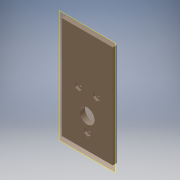
# Autodesk Inventor part: Motor cover lower
Saved by Autodesk Inventor 2019 (Build 230136000, 136)
## iProperties
Created: 2018-11-25
Part Number: Motor cover lower
Material: Generic
Document SubType Name: Modeling
Designer: Varga Daniel
Density: 1 g/cm^3
Appearance: Default
Author: Varga Daniel
Autodesk Inventor part; units mm, degrees
ref_plane "YZ Plane" through (0, 0, 0) normal (1, 0, 0) x (0, 1, 0)
ref_plane "XZ Plane" through (0, 0, 0) normal (0, 1, 0) x (-1, 0, 0)
ref_plane "Work Plane2" through (20, -5.2, 6) normal (0, 0, 1) x (1, 0, 0)
sketch "Sketch1" plane through (20, -5.2, 6) normal (0, 0, 1) x (1, 0, 0)
  line L0 (-33.75, 50) -> (16.25, 50)
  line L1 (16.25, 50) -> (16.25, -50)
  line L2 (16.25, -50) -> (-33.75, -50)
  line L3 (-33.75, -50) -> (-33.75, 50)
  line L4 (-33.75, 0) -> (16.25, 0) construction
  line L5 (-8.75, 50) -> (-8.75, -50) construction
  line L6 (-33.75, 0) -> (16.25, 0) construction
  circle A0 centre (-17.5, 0) radius 1.35
  circle A1 centre (0, 0) radius 1.35
  circle A2 centre (-8.75, -34.3) radius 1.35
  circle A3 centre (-8.75, -20.6) radius 7.25
  dimension "d0" = 50
  dimension "d1" = 100
  dimension "d15" = 2.7
  dimension "d16" = 2.7
  dimension "d17" = 2.7
  dimension "d18" = 14.5
  dimension "d19" = 17.5
  dimension "d20" = 20.6
  dimension "d21" = 34.3
  dimension "d22" = 15.7
  dimension "d23" = 16.25
  constraints: 14 end point, 6 midpoint, 4 centre point, 4 point on line, 2 parallel, 2 perpendicular, 1 horizontal
  measures "d0" distance between parallel lines of L3 L1
  measures "d1" distance between parallel lines of L2 L0
  measures "d15" diameter of A0
  measures "d16" diameter of A1
  measures "d17" diameter of A2
  measures "d18" diameter of A3
  measures "d19" distance of A1.centre A0.centre
  measures "d20" vertical distance of A3.centre A0.centre
  measures "d21" vertical distance of A2.centre A0.centre
  measures "d22" distance from line of A2.centre L2
  measures "d23" distance from line of A0.centre L3
extrude "Extrusion2" add sketch "Sketch1" against normal blind 4
sketch "Sketch2" plane through (20, -5.2, 6) normal (0, 0, 1) x (1, 0, 0)
  circle A0 centre (-8.75, -20.6) radius 7.25 construction
  circle A1 centre (-8.75, -34.3) radius 1.35 construction
  circle A2 centre (0, 0) radius 1.35 construction
  circle A3 centre (-17.5, 0) radius 1.35 construction
  line L0 (-33.75, 50) -> (16.25, 50) construction
  line L1 (-33.75, -50) -> (-33.75, 50) construction
  line L2 (16.25, -50) -> (-33.75, -50) construction
  line L3 (16.25, 50) -> (16.25, -50) construction
  line L4 (-14.4, -1.7898) -> (-17.5, -3.5796)
  line L5 (-17.5, -3.5796) -> (-20.6, -1.7898)
  line L6 (-20.6, -1.7898) -> (-20.6, 1.7898)
  line L7 (-20.6, 1.7898) -> (-17.5, 3.5796)
  line L8 (-17.5, 3.5796) -> (-14.4, 1.7898)
  line L9 (-14.4, 1.7898) -> (-14.4, -1.7898)
  line L10 (3.1, -1.7898) -> (0, -3.5796)
  line L11 (0, -3.5796) -> (-3.1, -1.7898)
  line L12 (-3.1, -1.7898) -> (-3.1, 1.7898)
  line L13 (-3.1, 1.7898) -> (0, 3.5796)
  line L14 (0, 3.5796) -> (3.1, 1.7898)
  line L15 (3.1, 1.7898) -> (3.1, -1.7898)
  line L16 (-5.65, -36.0898) -> (-8.75, -37.8796)
  line L17 (-8.75, -37.8796) -> (-11.85, -36.0898)
  line L18 (-11.85, -36.0898) -> (-11.85, -32.5102)
  line L19 (-11.85, -32.5102) -> (-8.75, -30.7204)
  line L20 (-8.75, -30.7204) -> (-5.65, -32.5102)
  line L21 (-5.65, -32.5102) -> (-5.65, -36.0898)
  line L22 (-33.75, -50) -> (-33.75, 50) projected
  point P0 (-20, 5.2)
  dimension "d26" = 6.2
  dimension "d27" = 6.2
  dimension "d28" = 6.2
  constraints: 36 end point, 3 coincident, 3 parallel, 39 other
  measures "d26" distance between parallel lines of L9 L6
  measures "d27" distance between parallel lines of L15 L12
  measures "d28" distance between parallel lines of L18 L21
extrude "Extrusion3" cut sketch "Sketch2" against normal blind 2.3
sketch "Sketch3" plane through (20, -5.2, 2) normal (0, 0, -1) x (-1, 0, 0)
  line L0 (19.7, 4.9) -> (-2.2, 4.9) construction
  line L1 (19.7, -28.8) -> (19.7, 4.9) construction
  arc A0 (17, -31.5) -> (19.7, -28.8) centre (17, -28.8) ccw construction
  line L2 (0.5, -31.5) -> (17, -31.5) construction
  arc A1 (-2.2, -28.8) -> (0.5, -31.5) centre (0.5, -28.8) ccw construction
  line L3 (-2.2, 4.9) -> (-2.2, -28.8) construction
  circle A2 centre (17.5, 0) radius 1.4 construction
  circle A3 centre (0, 0) radius 1.4 construction
  circle A4 centre (8.75, -9.4404) radius 2.05 construction
  circle A5 centre (8.85, -20.6) radius 2.8 construction
  arc A6 (-2.7, -28.8) -> (0.5, -32) centre (0.5, -28.8) ccw
  line L4 (0.5, -32) -> (17, -32)
  arc A7 (17, -32) -> (20.2, -28.8) centre (17, -28.8) ccw
  line L5 (20.2, -28.8) -> (20.2, 5.4)
  line L6 (20.2, 5.4) -> (-2.7, 5.4)
  line L7 (-2.7, 5.4) -> (-2.7, -28.8)
  circle A8 centre (0, 0) radius 1.9
  circle A9 centre (17.5, 0) radius 1.9
  circle A10 centre (8.75, -9.4404) radius 2.55
  circle A11 centre (8.75, -20.6) radius 7.25 construction
  circle A12 centre (8.75, -20.6) radius 7.75
  point P0 (20, 5.2)
  dimension "d31" = 0.5
  dimension "d32" = 0.5
  dimension "d33" = 0.5
  dimension "d34" = 0.5
  dimension "d35" = 0.5
  constraints: 8 end point, 6 centre point, 4 point on circle, 5 other
  measures "d31" distance between parallel lines of L3 L7
  measures "d32" radial gap between concentric circles of A3 A8
  measures "d33" radial gap between concentric circles of A2 A9
  measures "d34" radial gap between concentric circles of A4 A10
  measures "d35" radial gap between concentric circles of A11 A12
ref_plane "Work Plane3" through (0.3, -36.7, 0.5) normal (0, 0, 1) x (1, 0, 0)
extrude "Extrusion4" add sketch "Sketch3" along normal up to surface (1.5 mm away)
equation "\"d16\" = d15"
equation "\"d17\" = d15"
equation "\"d27\" = d26"
equation "\"d28\" = d26"
equation "\"d32\" = d31"
equation "\"d33\" = d31"
equation "\"d34\" = d31"
equation "\"d35\" = d31"
body "Solid2"
